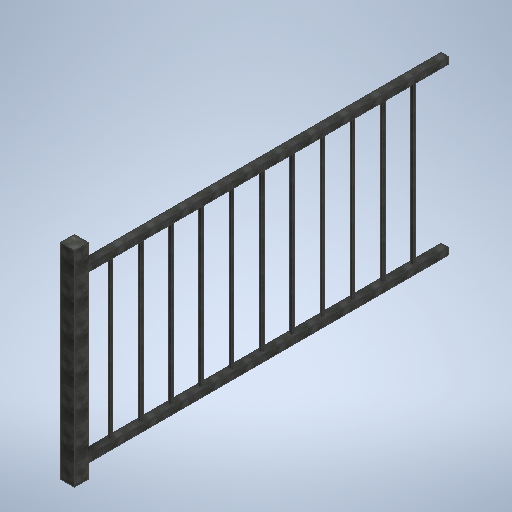
# Autodesk Inventor part: Railing
Saved by Autodesk Inventor 2025 (Build 290162000, 162)
## iProperties
Created: 2024-06-26
Part Number: Railing
Material: Iron, Wrought
Document SubType Name: Modeling
Designer: track
Density: 7.84905 g/cm^3
Appearance: Plate
Author: track
Autodesk Inventor part; units mm, degrees
ref_plane "YZ Plane" through (0, 0, 0) normal (1, 0, 0) x (0, 1, 0)
ref_plane "XZ Plane" through (0, 0, 0) normal (0, 1, 0) x (-1, 0, 0)
ref_plane "XY Plane" through (0, 0, 0) normal (0, 0, 1) x (1, 0, 0)
sketch "Sketch1" plane through (889, 0, -4876.8) normal (0, 1, 0) x (-1, 0, 0)
  line L0 (1778, 0) -> (1778, 9753.6)
  line L1 (1778, 0) -> (1701.8, 0)
  line L2 (1701.8, 0) -> (1701.8, 76.2)
  line L3 (1701.8, 76.2) -> (1778, 76.2)
  line L4 (1778, 76.2) -> (1778, 0)
  line L5 (889, 0) -> (889, 9753.6) construction
  line L6 (0, 9753.6) -> (1778, 9753.6)
  point P0 (0, 0)
  dimension "d0" = 76.2
  dimension "d1" = 76.2
  constraints: 14 end point, 2 parallel, 1 horizontal, 1 midpoint, 1 perpendicular
  measures "d0" distance of L2.end L3.end
  measures "d1" distance of L1.end L2.end
extrude "Extrusion1" add sketch "Sketch1" along normal blind 1117.6
sketch "Sketch2" plane through (-812.8, 0, -4876.8) normal (0, 0, -1) x (-1, 0, 0)
  line L0 (19.05, 95.25) -> (57.15, 95.25)
  line L1 (57.15, 95.25) -> (57.15, 57.15)
  line L2 (57.15, 57.15) -> (19.05, 57.15)
  line L3 (19.05, 57.15) -> (19.05, 95.25)
  line L4 (19.05, 95.25) -> (57.15, 57.15) construction
  line L5 (57.15, 95.25) -> (19.05, 57.15) construction
  line L6 (19.05, 996.95) -> (57.15, 996.95)
  line L7 (57.15, 996.95) -> (57.15, 958.85)
  line L8 (57.15, 958.85) -> (19.05, 958.85)
  line L9 (19.05, 958.85) -> (19.05, 996.95)
  line L10 (19.05, 996.95) -> (57.15, 958.85) construction
  line L11 (57.15, 996.95) -> (19.05, 958.85) construction
  line L12 (76.2, 55.9997) -> (76.2, 1188.6397)
  line L13 (76.2, 0) -> (76.2, 1117.6) projected
  line L14 (0, 0) -> (76.2, 0) projected
  point P0 (-812.8, 0)
  point P1 (64.1185, -20.2003)
  point P2 (38.1, 76.2)
  point P3 (38.1, 977.9)
  dimension "d5" = 38.1
  dimension "d6" = 38.1
  dimension "d7" = 38.1
  dimension "d9" = 863.6
  dimension "d10" = 38.1
  dimension "d11" = 38.1
  dimension "d12" = 38.1
  dimension "d13" = 76.2
  constraints: 26 end point, 4 midpoint, 4 parallel, 2 horizontal, 2 perpendicular, 1 point on line, 1 vertical
  measures "d5" distance of L0.end L1.end
  measures "d6" distance of L0.start L0.end
  measures "d7" distance from line of L12 point (38.1, 76.2)
  measures "d9" distance between parallel lines of L8 L0
  measures "d10" distance of L6.end L7.end
  measures "d11" distance of L6.start L6.end
  measures "d12" distance from line of L13 point (38.1, 977.9)
  measures "d13" distance from line of L14 point (38.1, 76.2)
extrude "Extrusion2" add sketch "Sketch2" along normal blind 1981.2
sketch "Sketch3" plane through (-831.85, 95.25, -4876.8) normal (0, 1, 0) x (1, 0, 0)
  line L0 (-19.05, 7.9484) -> (-19.05, 1981.2) construction
  line L1 (345.7063, 1981.2) -> (-383.8063, 1981.2)
  line L2 (-12.7, 152.4) -> (-25.4, 152.4)
  line L3 (-25.4, 152.4) -> (-25.4, 165.1)
  line L4 (-25.4, 165.1) -> (-12.7, 165.1)
  line L5 (-12.7, 165.1) -> (-12.7, 152.4)
  line L6 (-12.7, 152.4) -> (-25.4, 165.1) construction
  line L7 (-25.4, 152.4) -> (-12.7, 165.1) construction
  line L8 (-25.4, 317.5) -> (-25.4, 330.2)
  line L9 (-25.4, 330.2) -> (-12.7, 330.2)
  line L10 (-12.7, 330.2) -> (-12.7, 317.5)
  line L11 (-12.7, 317.5) -> (-25.4, 317.5)
  line L12 (-25.4, 482.6) -> (-25.4, 495.3)
  line L13 (-25.4, 495.3) -> (-12.7, 495.3)
  line L14 (-12.7, 495.3) -> (-12.7, 482.6)
  line L15 (-12.7, 482.6) -> (-25.4, 482.6)
  line L16 (-25.4, 647.7) -> (-25.4, 660.4)
  line L17 (-25.4, 660.4) -> (-12.7, 660.4)
  line L18 (-12.7, 660.4) -> (-12.7, 647.7)
  line L19 (-12.7, 647.7) -> (-25.4, 647.7)
  line L20 (-25.4, 812.8) -> (-25.4, 825.5)
  line L21 (-25.4, 825.5) -> (-12.7, 825.5)
  line L22 (-12.7, 825.5) -> (-12.7, 812.8)
  line L23 (-12.7, 812.8) -> (-25.4, 812.8)
  line L24 (-25.4, 977.9) -> (-25.4, 990.6)
  line L25 (-25.4, 990.6) -> (-12.7, 990.6)
  line L26 (-12.7, 990.6) -> (-12.7, 977.9)
  line L27 (-12.7, 977.9) -> (-25.4, 977.9)
  line L28 (-25.4, 1143) -> (-25.4, 1155.7)
  line L29 (-25.4, 1155.7) -> (-12.7, 1155.7)
  line L30 (-12.7, 1155.7) -> (-12.7, 1143)
  line L31 (-12.7, 1143) -> (-25.4, 1143)
  line L32 (-25.4, 1308.1) -> (-25.4, 1320.8)
  line L33 (-25.4, 1320.8) -> (-12.7, 1320.8)
  line L34 (-12.7, 1320.8) -> (-12.7, 1308.1)
  line L35 (-12.7, 1308.1) -> (-25.4, 1308.1)
  line L36 (-25.4, 1473.2) -> (-25.4, 1485.9)
  line L37 (-25.4, 1485.9) -> (-12.7, 1485.9)
  line L38 (-12.7, 1485.9) -> (-12.7, 1473.2)
  line L39 (-12.7, 1473.2) -> (-25.4, 1473.2)
  line L40 (-25.4, 1638.3) -> (-25.4, 1651)
  line L41 (-25.4, 1651) -> (-12.7, 1651)
  line L42 (-12.7, 1651) -> (-12.7, 1638.3)
  line L43 (-12.7, 1638.3) -> (-25.4, 1638.3)
  line L44 (-25.4, 1803.4) -> (-25.4, 1816.1)
  line L45 (-25.4, 1816.1) -> (-12.7, 1816.1)
  line L46 (-12.7, 1816.1) -> (-12.7, 1803.4)
  line L47 (-12.7, 1803.4) -> (-25.4, 1803.4)
  line L48 (19.05, 0) -> (-57.15, 0) projected
  line L49 (-38.1, 0) -> (-38.1, 1981.2) projected
  line L50 (-38.1, 1981.2) -> (0, 1981.2) projected
  point P0 (831.85, -4876.8)
  point P1 (-524.2437, -132.1024)
  point P2 (-19.05, 158.75)
  dimension "d20" = 12.7
  dimension "d21" = 12.7
  dimension "d23" = 165.1
  dimension "d25" = 152.4
  dimension "d27" = 19.05
  dimension "d28" = 0
  constraints: 96 end point, 3 midpoint, 2 parallel, 2 vertical, 1 horizontal, 1 perpendicular, 1 point on line, 80 other
  measures "d20" distance of L2.start L2.end
  measures "d21" distance of L4.end L2.start
  measures "d23" distance of L2.end L8.start
  measures "d25" distance between parallel lines of L48 L2
  measures "d27" distance between parallel lines of L49 L0
  measures "d28" distance between parallel lines of L50 L1
extrude "Extrusion3" add sketch "Sketch3" along normal up to surface (863.6 mm away)
body "Solid1"
